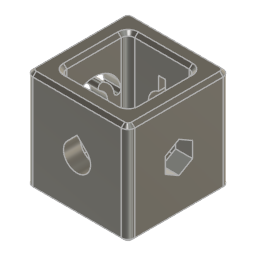
Hole Examples (Autodesk Fusion 360 design; units mm, degrees)
Autodesk Fusion 360 part; units mm, degrees
box "BoxPrimitive1" add length 30 width 30 height 30 placed x (0, 1, 0) y (-1, 0, 0) z (0, 0, 1) at (30, 0, 0)
shell "Shell1" thickness 5 removed faces 1 at (10, 10, 30)
sketch "Sketch2" plane through (0, 0, 0) normal (0, -1, 0) x (1, 0, 0)
  line L0 (0, 30) -> (0, 0)
  line L1 (0, 0) -> (30, 0)
  line L2 (30, 0) -> (30, 30)
  line L3 (30, 30) -> (0, 30)
  line L4 (0, 15) -> (30, 15) construction
  circle A0 centre (15, 15) radius 4
  line L5 (15, 15) -> (15, 20.6569) construction
  line L6 (15, 20.6569) -> (12.1716, 17.8284)
  line L7 (15, 20.6569) -> (17.8284, 17.8284)
  dimension "d9" = 8
  constraint midpoint L0 L4.start
  constraint midpoint L2 L4.end
  constraint midpoint L4 A0.centre
  constraint coincident A0.centre L5.start
  constraint perpendicular L4 L5
  constraint coincident A0 L6.end
  constraint tangent A0 L6
  constraint coincident A0 L7.end
  constraint perpendicular L6 L7
  constraint tangent A0 L7
  measures "d9" diameter of A0
extrude "Extrude1" cut sketch "Sketch2" against normal up to surface (5 mm away) contours A0 | A0 L6 L7
sketch "Sketch3" plane through (30, 0, 0) normal (1, 0, 0) x (0, 1, 0)
  line L0 (0, 30) -> (0, 0)
  line L1 (0, 0) -> (30, 0)
  line L2 (30, 0) -> (30, 30)
  line L3 (30, 30) -> (0, 30)
  line L4 (0, 15) -> (30, 15) construction
  line L5 (11, 17.3094) -> (11, 12.6906)
  line L6 (11, 12.6906) -> (15, 10.3812)
  line L7 (15, 10.3812) -> (19, 12.6906)
  line L8 (19, 12.6906) -> (19, 17.3094)
  line L9 (19, 17.3094) -> (15, 19.6188)
  line L10 (15, 19.6188) -> (11, 17.3094)
  point P0 (15, 15)
  dimension "d20" = 8
  constraint midpoint L0 L4.start
  constraint midpoint L2 L4.end
  constraint midpoint L4 P0
  constraint vertical L8
  measures "d20" distance of L7 L10
extrude "Extrude2" cut sketch "Sketch3" against normal up to surface (5 mm away) contours L5 L6 L7 L8 L9 L10
sketch "Sketch4" plane through (0, 30, 0) normal (0, 1, 0) x (-1, 0, 0)
  line L0 (-30, 30) -> (-30, 0)
  line L1 (-30, 0) -> (0, 0)
  line L2 (0, 0) -> (0, 30)
  line L3 (0, 30) -> (-30, 30)
  line L4 (-30, 15) -> (0, 15) construction
  circle A0 centre (-15, 15) radius 4
  line L5 (-15, 15) -> (-15, 19) construction
  line L6 (-16, 18.873) -> (-16, 22.873)
  line L7 (-14, 18.873) -> (-14, 22.873)
  line L8 (-16, 22.873) -> (-14, 22.873)
  line L9 (-16, 11.127) -> (-16, 7.127)
  line L10 (-16, 7.127) -> (-14, 7.127)
  line L11 (-14, 11.127) -> (-14, 7.127)
  dimension "d15" = 8
  dimension "d16" = 2
  dimension "d17" = 4
  constraint midpoint L0 L4.start
  constraint midpoint L2 L4.end
  constraint midpoint L4 A0.centre
  constraint coincident A0.centre L5.start
  constraint perpendicular L4 L5
  constraint coincident A0 L6.start
  constraint vertical L6
  constraint symmetric L5 L6.start L7.start
  constraint symmetric L5 L6.end L7.end
  constraint symmetric L4 L6.start L9.start
  constraint symmetric L4 L6.end L9.end
  constraint symmetric L4 L7.start L11.start
  constraint symmetric L4 L7.end L10.end
  measures "d15" diameter of A0
  measures "d16" distance of L9.end L10.end
  measures "d17" distance of L10.end L11.start
extrude "Extrude3" cut sketch "Sketch4" against normal up to surface (5 mm away) contours A0 | A0 L6 L7 L8 | A0 L9 L10 L11
sketch "Sketch5" plane through (0, 0, 0) normal (-1, 0, 0) x (0, -1, 0)
  line L0 (-30, 30) -> (-30, 0)
  line L1 (-30, 0) -> (0, 0)
  line L2 (0, 0) -> (0, 30)
  line L3 (0, 30) -> (-30, 30)
  line L4 (-30, 15) -> (0, 15) construction
  circle A0 centre (-15, 15) radius 4
  arc A1 (-7.0821, 16.1429) -> (-22.9179, 16.1429) centre (-15, 15) ccw
  arc A2 (-9.0615, 15.8571) -> (-7.0821, 16.1429) centre (-8.0718, 16) ccw
  arc A3 (-9.0615, 15.8571) -> (-20.9385, 15.8571) centre (-15, 15) ccw
  arc A4 (-22.9179, 16.1429) -> (-20.9385, 15.8571) centre (-21.9282, 16) ccw
  arc A5 (-8.0718, 16) -> (-21.9282, 16) centre (-15, 15) ccw construction
  line L5 (-15, 15) -> (-15, 21.8872) construction
  line L6 (-15, 15) -> (-16.5529, 20.7956) construction
  arc A6 (-16.7871, 18.5786) -> (-17.6806, 20.3679) centre (-17.2339, 19.4732) ccw
  arc A7 (-12.3194, 20.3679) -> (-13.2129, 18.5786) centre (-12.7661, 19.4732) ccw
  line L7 (-15, 15) -> (-17.6806, 20.3679) construction
  dimension "d21" = 8
  dimension "d22" = 2
  dimension "d23" = 2
  dimension "d24" = 1
  dimension "d25" = 15
  dimension "d26" = 1
  constraint midpoint L0 L4.start
  constraint midpoint L2 L4.end
  constraint midpoint L4 A0.centre
  constraint tangent A1 A2
  constraint tangent A2 A3
  constraint tangent A3 A4
  constraint tangent A1 A4
  constraint coincident A0.centre A1.centre
  constraint horizontal A4.centre A2.centre
  constraint perpendicular L4 L5
  constraint coincident A3 L6.end
  constraint tangent L6 A6
  constraint coincident A0 A6.start
  constraint coincident A3 A6.end
  constraint symmetric L5 A6.end A7.start
  constraint symmetric L5 A6.start A7.end
  constraint symmetric L5 A6 A7
  constraint coincident A6.end L7.end
  measures "d21" diameter of A0
  measures "d22" distance of A0 A3
  measures "d23" distance of A1 A3
  measures "d24" distance of L4 A4.centre
  measures "d25" angle of L5 L6
  measures "d26" distance of L6 A6.centre
extrude "Extrude4" cut sketch "Sketch5" against normal up to surface (5 mm away) contours A0 | A0 A3 A6 A7 | A1 A2 A3 A4
fillet "Fillet1" radius 2 8 edges at (0, 30, 15) (0, 0, 15) (30, 0, 15) (30, 30, 15) (25, 5, 17.5) (5, 5, 17.5) (5, 25, 17.5) (25, 25, 17.5)
sketch "Sketch6" plane through (0, 0, 0) normal (0, 0, -1) x (1, 0, 0)
  arc A0 (28, -30) -> (30, -28) centre (28, -28) ccw
  line L0 (30, -28) -> (30, -2)
  arc A1 (30, -2) -> (28, 0) centre (28, -2) ccw
  line L1 (28, 0) -> (2, 0)
  arc A2 (2, 0) -> (0, -2) centre (2, -2) ccw
  line L2 (0, -2) -> (0, -28)
  arc A3 (0, -28) -> (2, -30) centre (2, -28) ccw
  line L3 (2, -30) -> (28, -30)
  line L4 (30, -15) -> (0, -15) construction
  circle A4 centre (15, -15) radius 4
  dimension "d31" = 8
  constraint midpoint L0 L4.start
  constraint midpoint L2 L4.end
  constraint midpoint L4 A4.centre
  measures "d31" diameter of A4
extrude "Extrude5" cut sketch "Sketch6" against normal up to surface (5 mm away) contours A4
chamfer "Chamfer1" distance 1 angle 45 24 edges at (30, 15, 30) (29.4142, 29.4142, 30) (15, 30, 30) (0.5858, 29.4142, 30) (0, 15, 30) (0.5858, 0.5858, 30) (15, 0, 30) (29.4142, 0.5858, 30) (15, 0, 0) (0.5858, 0.5858, 0) (0, 15, 0) (0.5858, 29.4142, 0) (15, 30, 0) (29.4142, 29.4142, 0) (30, 15, 0) (29.4142, 0.5858, 0) (25, 15, 30) (24.4142, 5.5858, 30) (15, 5, 30) (5.5858, 5.5858, 30) (5, 15, 30) (5.5858, 24.4142, 30) (15, 25, 30) (24.4142, 24.4142, 30)
equation "d9 = HoleDiameter"
equation "d15 = HoleDiameter"
equation "d20 = HoleDiameter"
equation "d21 = HoleDiameter"
equation "d26 = d22 / 2"
equation "d31 = HoleDiameter"
equation "HoleDiameter = 8 mm"
named bodies: "Hole Examples"
